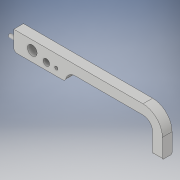
# Autodesk Inventor part: BRAZO BALSA UNDIMOTRIZ
Saved by Autodesk Inventor 2019.4 (Build 234330000, 330)
## iProperties
Created: 2020-08-23
Part Number: BRAZO BALSA UNDIMOTRIZ
Material: Generic
Document SubType Name: Modeling
Designer: crist
Density: 1 g/cm^3
Appearance: Default
Author: crist
Autodesk Inventor part; units mm, degrees
ref_plane "YZ Plane" through (0, 0, 0) normal (1, 0, 0) x (0, 1, 0)
ref_plane "XZ Plane" through (0, 0, 0) normal (0, 1, 0) x (-1, 0, 0)
ref_plane "XY Plane" through (0, 0, 0) normal (0, 0, 1) x (1, 0, 0)
sketch "Boceto1" plane through (0, 0, 0) normal (0, 0, 1) x (1, 0, 0)
  arc A0 (1500, 0) -> (0, 1500) centre (0, 0) ccw
  arc A1 (3000, 0) -> (0, 3000) centre (0, 0) ccw
  line L0 (3000, 0) -> (3000, -3000)
  line L1 (3000, -3000) -> (1500, -3000)
  line L2 (1500, -3000) -> (1500, 0)
  line L3 (0, 3000) -> (-20000, 3000)
  line L4 (-20000, 3000) -> (-20000, 0)
  line L5 (-20000, 0) -> (-12000, 0)
  arc A2 (-10500, 1500) -> (-12000, 0) centre (-10500, 0) ccw
  line L6 (0, 1500) -> (-10500, 1500)
  dimension "d4" = 3000
  dimension "d5" = 6000
  dimension "d7" = 20000
  dimension "d8" = 8000
  dimension "d10" = 3000
  constraints: 14 end point, 6 point on circle, 4 perpendicular, 3 centre point, 2 coincident, 2 horizontal, 1 vertical
  measures "d4" diameter of A0
  measures "d5" diameter of A1
  measures "d7" distance of L3.start L3.end
  measures "d8" distance of L4.end L5.end
  measures "d10" distance of L0.start L0.end
extrude "Extrusión1" add sketch "Boceto1" along normal blind 1500
fillet "Empalme1" radius 500 1 edges at (-12000, 0, 750)
sketch "Boceto2" plane through (0, 0, 1500) normal (0, 0, 1) x (1, 0, 0)
  circle A0 centre (-13410.7545, 1088.9074) radius 250
  circle A1 centre (-14953.0607, 1088.9074) radius 500
  circle A2 centre (-17138.5672, 1588.9074) radius 750
  point P0 (0, 0)
  dimension "d14" = 500
  dimension "d15" = 1000
  dimension "d16" = 1500
  constraints: 3 centre point
  measures "d14" diameter of A0
  measures "d15" diameter of A1
  measures "d16" diameter of A2
extrude "Extrusión2" cut sketch "Boceto2" against normal blind 1500
fillet "Empalme2" radius 500 1 edges at (-20000, 0, 750)
fillet "Empalme3" radius 200 1 edges at (2250, -3000, 1500)
fillet "Empalme4" radius 200 1 edges at (2250, -3000, 0)
sketch "Boceto3" plane through (-20000, 3000, 0) normal (-1, 0, 0) x (0, 0, 1)
  circle A0 centre (300, -1411.0926) radius 250
  circle A1 centre (1200, -1411.0926) radius 250
  point P0 (0, -3000)
  dimension "d24" = 500
  dimension "d26" = 500
  constraints: 2 centre point
  measures "d24" diameter of A0
  measures "d26" diameter of A1
extrude "Extrusión3" add sketch "Boceto3" along normal blind 900
